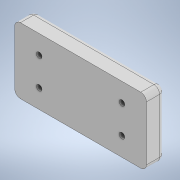
# Autodesk Inventor part: Peça4-Rubia
Saved by Autodesk Inventor 2021 (Build 250183000, 183)
## iProperties
Created: 2021-03-18
Part Number: Peça4-Rubia
Material: Genérico
Document SubType Name: Modeling
Designer: rubia
Density: 1 g/cm^3
Appearance: Padrão
Author: rubia
Autodesk Inventor part; units mm, degrees
ref_plane "YZ Plane" through (0, 0, 0) normal (1, 0, 0) x (0, 1, 0)
ref_plane "XZ Plane" through (0, 0, 0) normal (0, 1, 0) x (-1, 0, 0)
ref_plane "XY Plane" through (0, 0, 0) normal (0, 0, 1) x (1, 0, 0)
sketch "Esboço1" plane through (0, 0, 0) normal (0, 0, 1) x (1, 0, 0)
  line L0 (0, 0) -> (70, 0)
  line L1 (70, 0) -> (70, 35)
  line L2 (70, 35) -> (0, 35)
  line L3 (0, 35) -> (0, 0)
  dimension "d0" = 70
  dimension "d1" = 35
  constraints: 8 end point, 2 parallel, 1 horizontal, 1 perpendicular
  measures "d0" distance of L2.end L1.end
  measures "d1" distance of L1.end L0.end
extrude "Extrusão1" add sketch "Esboço1" along normal blind 10
fillet "Arredondamento1" radius 3 4 edges at (70, 35, 5) (70, 0, 5) (0, 35, 5) (0, 0, 5)
fillet "Arredondamento2" radius 3 8 edges at (0.8787, 34.1213, 0) (0, 17.5, 0) (0.8787, 0.8787, 0) (35, 0, 0) (69.1213, 0.8787, 0) (70, 17.5, 0) (69.1213, 34.1213, 0) (35, 35, 0)
sketch "Esboço3" plane through (0, 0, 0) normal (0, 0, -1) x (-1, 0, 0)
  line L0 (-3, 35) -> (-67, 35) projected
  line L1 (-67, 3) -> (-67, 32) projected
  line L2 (-67, 0) -> (-3, 0) projected
  line L3 (-3, 32) -> (-3, 3) projected
  point P0 (0, 0)
  point P1 (-57, 25)
  point P2 (-13, 25)
  point P3 (-13, 10)
  point P4 (-57, 10)
  dimension "d18" = 10
  dimension "d19" = 10
  dimension "d20" = 10
  dimension "d21" = 10
  dimension "d22" = 10
  dimension "d23" = 10
  dimension "d24" = 10
  dimension "d25" = 10
  measures "d18" distance from line of L0 point (-57, 25)
  measures "d19" distance from line of L1 point (-57, 25)
  measures "d20" distance from line of L2 point (-57, 10)
  measures "d21" distance from line of L1 point (-57, 10)
  measures "d22" distance from line of L0 point (-13, 25)
  measures "d23" distance from line of L3 point (-13, 25)
  measures "d24" distance from line of L3 point (-13, 10)
  measures "d25" distance from line of L2 point (-13, 10)
hole "Furo1" at (57, 25, 0) at (13, 25, 0) at (13, 10, 0) at (57, 10, 0) direction (0, 0, 1) diameter 3 end through all
thread "Rosca1" size "M3x0.35" class "6H" standard "ANSI Metric M Profile" length 3 offset 7
thread "Rosca2" size "M3x0.5" class "6H" standard "ANSI Metric M Profile" length 3
thread "Rosca3" size "M3x0.5" class "6H" standard "ANSI Metric M Profile" length 3
thread "Rosca4" size "M3x0.5" class "6H" standard "ANSI Metric M Profile" length 3
equation "\"d19\" = d18"
equation "\"d20\" = d18"
equation "\"d21\" = d18"
equation "\"d22\" = d18"
equation "\"d23\" = d18"
equation "\"d24\" = d18"
equation "\"d25\" = d18"
